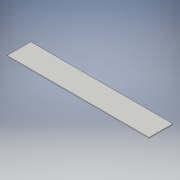
# Autodesk Inventor part: Shim1-32
Saved by Autodesk Inventor 2019 (Build 230136000, 136)
## iProperties
Created: 2019-02-11
Part Number: Shim1-32
Material: Generic
Document SubType Name: Modeling
Designer: james
Density: 1 g/cm^3
Appearance: Default
Author: james
Autodesk Inventor part; units mm, degrees
ref_plane "YZ Plane" through (0, 0, 0) normal (1, 0, 0) x (0, 1, 0)
ref_plane "XZ Plane" through (0, 0, 0) normal (0, 1, 0) x (-1, 0, 0)
ref_plane "XY Plane" through (0, 0, 0) normal (0, 0, 1) x (1, 0, 0)
sketch "Sketch1" plane through (0, 0, 0) normal (0, 1, 0) x (-1, 0, 0)
  line L0 (17.4625, 22.387) -> (-134.9375, 22.387)
  line L1 (-134.9375, 22.387) -> (-134.9375, -3.013)
  line L2 (-134.9375, -3.013) -> (17.4625, -3.013)
  line L3 (17.4625, -3.013) -> (17.4625, 22.387)
  point P0 (0, 0)
  dimension "d0" = 25.4
  dimension "d1" = 152.4
  constraints: 8 end point, 2 parallel, 1 horizontal, 1 perpendicular
  measures "d0" distance of L2.end L0.start
  measures "d1" distance of L1.end L2.end
extrude "Extrusion1" add sketch "Sketch1" along normal blind 0.7937
body "Solid1"
